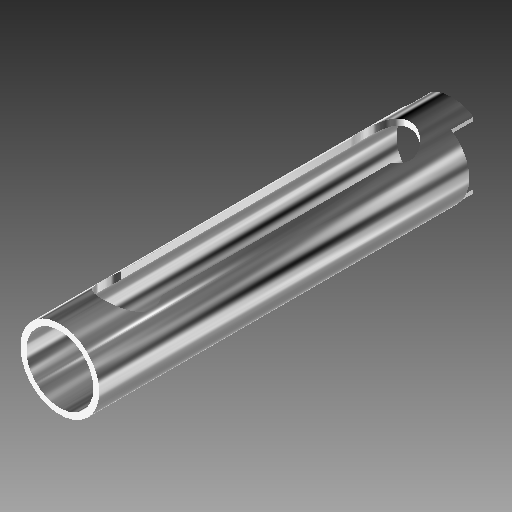
# Autodesk Inventor part: 308-13
Saved by Autodesk Inventor 2019 (Build 230136000, 136)
## iProperties
Company: Autodesk Inc.
Created: 2012-01-24
Part Number: 308-13
Material: Steel, Mild
Document SubType Name: Modeling
Designer: Autodesk Inc.
Mass: 3.4955 g
Surface Area: 15.6612 cm^2
Volume: 0.445287 cm^3
Density: 7.85 g/cm^3
Appearance: Chrome - Polished
Author: Inventor
Autodesk Inventor part; units mm, degrees
ref_plane "YZ Plane" through (0, 0, 0) normal (1, 0, 0) x (0, 1, 0)
sketch "Sketch1" plane through (0, 0, 0) normal (0, 0, 1) x (1, 0, 0)
  circle A0 centre (0, 0) radius 3.975
  circle A1 centre (0, 0) radius 3.375
  dimension "d0" = 7.95
  dimension "d1" = 0.6
  constraints: 2 centre point, 2 coincident
  measures "d0" diameter of A0
  measures "d1" radial gap between concentric circles of A0 A1
extrude "Extrusion1" add sketch "Sketch1" along normal blind 39.55
ref_plane "Work Plane1" through (0, -3.975, 0) normal (0, 1, 0) x (-1, 0, 0)
sketch "Sketch2" plane through (0, -3.975, 0) normal (0, 1, 0) x (-1, 0, 0)
  line L0 (0, 0) -> (0, 6.8) construction
  line L1 (0, 6.8) -> (0, 32.8) construction
  circle A0 centre (0, 32.8) radius 2.5
  circle A1 centre (0, 6.8) radius 2.5
  line L2 (2.075, 32.8) -> (-2.075, 32.8)
  line L3 (-2.075, 32.8) -> (-2.075, 6.8)
  line L4 (-2.075, 6.8) -> (2.075, 6.8)
  line L5 (2.075, 6.8) -> (2.075, 32.8)
  dimension "d4" = 6.8
  dimension "d5" = 26
  dimension "d6" = 5
  dimension "d7" = 4.15
  constraints: 12 end point, 2 centre point, 2 coincident, 2 midpoint, 2 parallel, 1 collinear, 1 equal radius, 1 horizontal, 1 perpendicular, 1 vertical
  measures "d4" distance of L0.start L0.end
  measures "d5" distance of L0.end L1.end
  measures "d6" diameter of A0
  measures "d7" distance of L3.end L4.end
extrude "Extrusion2" cut sketch "Sketch2" along normal up to surface
ref_plane "Work Plane2" through (0, 0, 37.3) normal (0, 0, -1) x (-1, 0, 0)
sketch "Sketch3" plane through (0, 0, 39.55) normal (0, 0, 1) x (1, 0, 0)
  circle A0 centre (0, 0) radius 3.375 projected
  circle A1 centre (0, 0) radius 3.975 projected
  line L0 (2.15, 4.5) -> (2.15, -4.5)
  line L1 (-2.15, -4.5) -> (-2.15, 4.5)
  line L2 (-2.15, 0) -> (2.15, 0) construction
  arc A2 (-2.15, 4.5) -> (-2.15, -4.5) centre (1.8186, 0) ccw
  arc A3 (2.15, -4.5) -> (2.15, 4.5) centre (-1.8186, 0) ccw
  point P0 (0, 0)
  dimension "d20" = 4.3
  dimension "d21" = 9
  dimension "d22" = 6
  dimension "d23" = 6
  constraints: 6 end point, 4 point on circle, 3 midpoint, 2 centre point, 2 parallel, 1 coincident, 1 horizontal alignment, 1 perpendicular
  measures "d20" distance of L1.end L0.start
  measures "d21" distance of L0.start L0.end
  measures "d22" radius of A2
  measures "d23" radius of A3
extrude "Extrusion3" cut sketch "Sketch3" against normal up to surface (2.25 mm away) contours A0 L0 | A0 L0 A1 | L1 A0 | A0 L1 A1 | L0 A3 A1 | A1 L1 A2
chamfer "Chamfer1" distance 0.25 distance2 0.75 2 edges at (0, -3.375, 39.55) (0, 3.375, 39.55) measured on face at (1.662, -3.3702, 39.55) measured on face at (1.662, 3.3702, 39.55)
chamfer "Chamfer2" distance 0.375 angle 45 4 edges at (2.15, -2.6016, 38.05) (2.15, 2.6016, 38.05) (-2.15, -2.6016, 38.05) (-2.15, 2.6016, 38.05)
body "Solid1"
